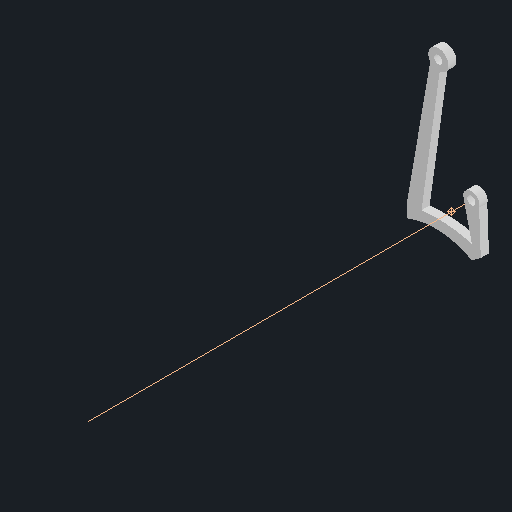
# Autodesk Inventor part: Trigger
Saved by Autodesk Inventor 2024.1 (Build 281209000, 209)
## iProperties
Created: 2023-08-21
Part Number: Trigger
Material: Generic
Document SubType Name: Modeling
Designer: Eleanor
Density: 1 g/cm^3
Appearance: Default
Author: Eleanor
Autodesk Inventor part; units mm, degrees
ref_plane "YZ Plane" through (0, 0, 0) normal (1, 0, 0) x (0, 1, 0)
ref_plane "XZ Plane" through (0, 0, 0) normal (0, 1, 0) x (-1, 0, 0)
ref_plane "XY Plane" through (0, 0, 0) normal (0, 0, 1) x (1, 0, 0)
sketch "Sketch2" plane through (0, 0, 0) normal (0, 0, 1) x (1, 0, 0)
  circle A0 centre (-10.9433, 29.4991) radius 1.5875
  arc A1 (-7.9093, 28.5632) -> (-13.7976, 28.1085) centre (-10.9433, 29.4991) ccw
  line L0 (-7.9093, 28.5632) -> (-7.2718, 11.9066)
  line L1 (-7.2718, 11.9066) -> (-10.7903, 9.3453)
  line L2 (-14.1183, 29.4991) -> (-10.7522, 14.9045)
  arc A2 (-10.7522, 14.9045) -> (-30.3533, 16.4875) centre (-24.5669, -34.0068) ccw
  arc A3 (-10.7903, 9.3453) -> (-36.1457, 10.8505) centre (-25.0332, -16.2685) ccw
  line L3 (0, 0) -> (-13.4011, 0)
  line L4 (0, 0) -> (0, 33.0147)
  line L5 (-36.1457, 15.4815) -> (-36.1457, 10.8505)
  line L6 (-36.1457, 15.4815) -> (-26.9875, 68.2625)
  line L7 (-30.3533, 16.4875) -> (-23.2965, 66.675)
  arc A4 (-23.2965, 66.675) -> (-26.9875, 68.2625) centre (-23.8136, 70.5573) ccw
  circle A5 centre (-23.8136, 70.5573) radius 1.5875
  dimension "d0" = 3.175
  dimension "d1" = 6.35
  dimension "d2" = 25.4
  dimension "d3" = 25.4
  dimension "d4" = 31.4635
  dimension "d5" = 10.9433
  dimension "d6" = 29.4991
  dimension "d7" = 4.631
  dimension "d8" = 5.5592
  dimension "d9" = 2.9979
  dimension "d11" = 17.7614
  constraints: 16 end point, 9 point on circle, 6 centre point, 3 coincident, 2 vertical, 1 horizontal, 1 point on line
  measures "d0" diameter of A0
  measures "d1" diameter of A1
  measures "d2" distance of L2.end L5.start
  measures "d3" distance of L1.end L5.end
  measures "d4" distance of L3.start A0.centre
  measures "d5" distance from line of L4 A0.centre
  measures "d6" distance from line of L3 A0.centre
  measures "d7" distance of L5.start L5.end
  measures "d8" vertical distance of L1.end L2.end
  measures "d9" vertical distance of L0.end L2.end
  measures "d11" horizontal distance of A3.centre L0.end
extrude "Extrusion1" add sketch "Sketch2" along normal blind 3.175 contours A0 | L0 L1 A3 L5 L6 A4 L7 A2 L2 A1 | A5
hole "Hole1" at (-10.9423, 29.498, 11.1125) direction (0, 0, -1) diameter 3.175 end through all
hole "Hole4" at (-10.9433, 29.4991, 0) at (-23.8136, 70.5573, 0) direction (0, 0, 1) diameter 3.175 depth 25.4 tip angle 118
body "Solid1"
